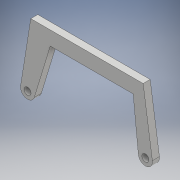
# Autodesk Inventor part: barra_c
Saved by Autodesk Inventor 2018 (Build 220112000, 112)
## iProperties
Created: 2018-05-25
Part Number: barra_c
Material: Generic
Document SubType Name: Modeling
Designer: vigus
Density: 1 g/cm^3
Appearance: Default
Author: vigus
Autodesk Inventor part; units mm, degrees
ref_plane "YZ Plane" through (0, 0, 0) normal (1, 0, 0) x (0, 1, 0)
ref_plane "XZ Plane" through (0, 0, 0) normal (0, 1, 0) x (-1, 0, 0)
ref_plane "XY Plane" through (0, 0, 0) normal (0, 0, 1) x (1, 0, 0)
sketch "Sketch1" plane through (0, 0, 0) normal (0, 1, 0) x (-1, 0, 0)
  circle A0 centre (26.0324, -0.4741) radius 1.5
  circle A1 centre (-24.2562, 0) radius 3
  circle A2 centre (-24.2562, 0) radius 1.5
  circle A3 centre (26.0324, -0.4741) radius 3
  line L0 (0, 0) -> (-28.1337, 0) construction
  line L1 (0, 0) -> (28.9947, 0) construction
  line L2 (28.9947, 0) -> (24.6719, 27.0084)
  line L3 (-23.6062, 24.8761) -> (-27.2238, 0.4393)
  line L4 (23.1627, -1.3485) -> (16.3374, 21.053)
  line L5 (16.3374, 21.053) -> (-19.0472, 21.053)
  line L6 (-19.0472, 21.053) -> (-21.2723, -0.3108)
  line L7 (24.6719, 27.0084) -> (-23.2906, 27.0084)
  line L8 (-23.2906, 27.0084) -> (-23.6062, 24.8761)
  dimension "d8" = 3
  dimension "d9" = 6
  dimension "d10" = 3
  dimension "d12" = 6
  dimension "d13" = 180
  constraints: 18 end point, 4 centre point, 4 point on circle, 4 tangent, 2 coincident, 2 horizontal, 1 collinear, 1 point on line
  measures "d8" diameter of A0
  measures "d9" diameter of A1
  measures "d10" diameter of A2
  measures "d12" diameter of A3
  measures "d13" angle of L0 L1
extrude "Extrusion1" add sketch "Sketch1" along normal blind 3
body "Solid1"
